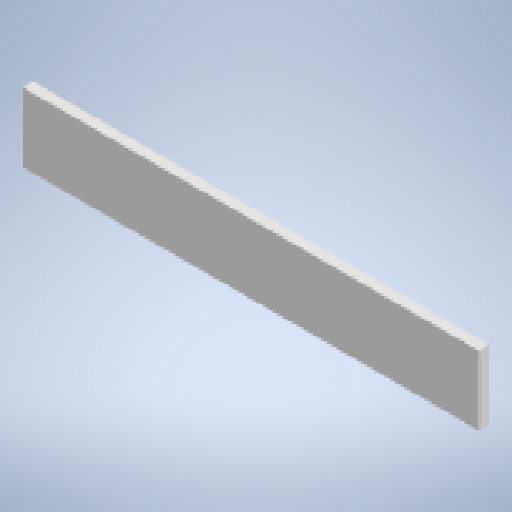
# Autodesk Inventor part: spacer
Saved by Autodesk Inventor 2023 (Build 270158000, 158)
## iProperties
Created: 2023-02-02
Part Number: spacer
Material: Generic
Document SubType Name: Modeling
Designer: shrey
Density: 1 g/cm^3
Appearance: Default
Author: shrey
Autodesk Inventor part; units mm, degrees
ref_plane "YZ Plane" through (0, 0, 0) normal (1, 0, 0) x (0, 1, 0)
ref_plane "XZ Plane" through (0, 0, 0) normal (0, 1, 0) x (-1, 0, 0)
ref_plane "XY Plane" through (0, 0, 0) normal (0, 0, 1) x (1, 0, 0)
sketch "Sketch1" plane through (0, 0, 0) normal (0, 0, 1) x (1, 0, 0)
  line L0 (-157.15, 140.4486) -> (-157.15, -171.5087) projected
  line L1 (-157.15, -171.5087) -> (157.15, -171.5087) projected
  line L2 (157.15, -171.5087) -> (157.15, 140.4486) projected
  line L3 (157.15, 140.4486) -> (-157.15, 140.4486) projected
  line L4 (66.075, 96.6673) -> (66.075, 141.6673) projected
  line L5 (66.075, 96.6673) -> (-66.075, 96.6673)
  line L6 (-66.075, 96.6673) -> (-66.075, 116.6673)
  line L7 (-66.075, 116.6673) -> (66.075, 116.6673)
  line L8 (66.075, 116.6673) -> (66.075, 96.6673)
  point P0 (0, 0)
  dimension "d0" = 132.15
  dimension "d1" = 20
  constraints: 8 end point, 2 parallel, 1 horizontal, 1 perpendicular
  measures "d0" distance of L6.end L7.end
  measures "d1" distance of L5.end L6.end
extrude "Extrusion1" add sketch "Sketch1" along normal blind 3 contours L5 L6 L7 L4
body "Solid1"
